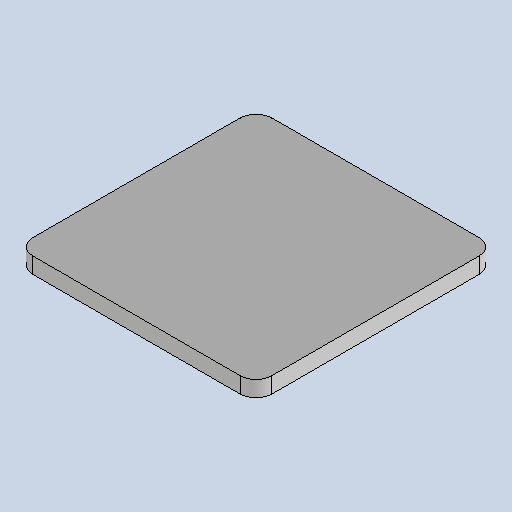
# Autodesk Inventor part: APN 766 FDS 1200 CUP 1
Saved by Autodesk Inventor 2025.1 (Build 291241020, 241B)
## iProperties
Created: 2025-06-24
Part Number: APN 766 FDS 1200 CUP 1
Material: Stainless Steel
Document SubType Name: Sheet Metal
Designer: user
Mass: 14.3451 g
Surface Area: 20.2627 cm^2
Volume: 1.79313 cm^3
Density: 8 g/cm^3
Flat Pattern Width: 3 cm
Flat Pattern Length: 3 cm
Flat Pattern Area: 9 cm^2
Sheet Metal Rule: AISI304 2mm Die16
Sheet Metal Width: 30.000 mm
Sheet Metal Length: 30.000 mm
Sheet Metal Area: 900.000 mm^2
Appearance: Default
Author: user
Autodesk Inventor part; units mm, degrees
ref_plane "YZ Plane" through (0, 0, 0) normal (1, 0, 0) x (0, 1, 0)
ref_plane "XZ Plane" through (0, 0, 0) normal (0, 1, 0) x (-1, 0, 0)
ref_plane "XY Plane" through (0, 0, 0) normal (0, 0, 1) x (1, 0, 0)
sketch "Sketch1" plane through (0, 0, 0) normal (0, 0, 1) x (1, 0, 0)
  line L0 (-15, -15) -> (15, -15)
  line L1 (15, -15) -> (15, 15)
  line L2 (15, 15) -> (-15, 15)
  line L3 (-15, 15) -> (-15, -15)
  line L4 (-15, -15) -> (15, 15) construction
  line L5 (15, -15) -> (-15, 15) construction
  point P0 (0, 0)
  dimension "d154" = 30
  dimension "d155" = 30
  measures "d154" distance of L1.end L2.end
  measures "d155" distance of L0.end L1.end
extrude "Plate5" add sketch "Sketch1" along normal blind 2
fillet "Corner Round1" radius 2 4 edges at (15, 15, 1) (-15, 15, 1) (-15, -15, 1) (15, -15, 1)
body "Solid3"
